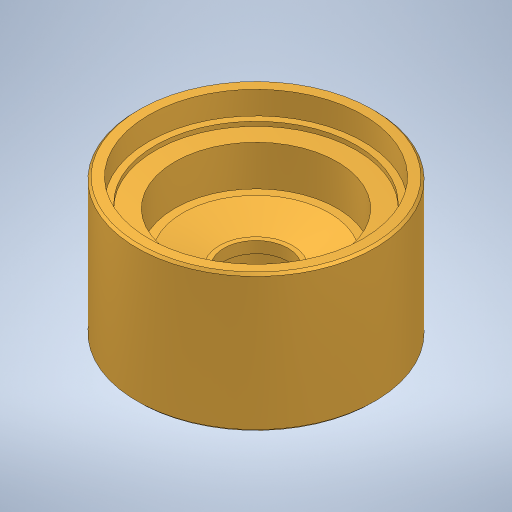
# Autodesk Inventor part: Flywheel
Saved by Autodesk Inventor 2023.2 (Build 272271000, 271)
## iProperties
Created: 2024-02-03
Part Number: Flywheel
Material: Brass, Soft Yellow
Document SubType Name: Modeling
Designer: Nathan Cai
Mass: 186.843 g
Surface Area: 85.7696 cm^2
Volume: 22.0594 cm^3
Density: 8.47 g/cm^3
Appearance: Brass - Satin
Author: Nathan Cai
Autodesk Inventor part; units mm, degrees
ref_plane "YZ Plane" through (0, 0, 0) normal (1, 0, 0) x (0, 1, 0)
ref_plane "XZ Plane" through (0, 0, 0) normal (0, 1, 0) x (-1, 0, 0)
ref_plane "XY Plane" through (0, 0, 0) normal (0, 0, 1) x (1, 0, 0)
sketch "Sketch2" plane through (0, 0, 0) normal (1, 0, 0) x (0, 1, 0)
  line L0 (0, 0) -> (19.05, 0)
  line L1 (19.05, 0) -> (19.05, -6.35)
  line L2 (19.05, -6.35) -> (0, -6.35)
  line L3 (0, -6.35) -> (0, 0)
  line L4 (0, 0) -> (19.05, 0)
  line L5 (19.05, 0) -> (19.05, -20.6375)
  line L6 (19.05, -20.6375) -> (0, -20.6375)
  line L7 (0, -20.6375) -> (0, 0)
  line L8 (0, -16.7624) -> (10.3188, -16.7624) construction
  line L9 (10.3188, -16.7624) -> (10.3188, -6.35)
  line L10 (10.3188, -6.35) -> (0, -6.35)
  line L11 (0, -6.35) -> (0, -16.7624)
  line L12 (10.3188, -16.7624) -> (0, -19.05)
  line L13 (6.35, -20.6375) -> (19.05, -17.4625)
  line L14 (19.05, 0) -> (12.05, 0)
  line L15 (12.05, 0) -> (12.05, -13.975)
  line L16 (12.05, -13.975) -> (19.05, -13.975)
  line L17 (19.05, -13.975) -> (19.05, 0)
  line L18 (10.3188, -15.0812) -> (4.7625, -15.0812)
  line L19 (4.7625, -15.0812) -> (4.7625, -6.35)
  line L20 (4.7625, -6.35) -> (10.3188, -6.35)
  line L21 (10.3188, -6.35) -> (10.3188, -15.0812)
  line L22 (4.7625, -9.525) -> (10.3188, -15.0812)
  line L23 (19.05, 0) -> (23.8125, 0)
  line L24 (23.8125, 0) -> (23.8125, -20.6375)
  line L25 (23.8125, -20.6375) -> (19.05, -20.6375)
  line L26 (19.05, -20.6375) -> (19.05, 0)
  line L27 (23.8125, 0) -> (19.8125, 0)
  line L28 (19.8125, 0) -> (19.8125, -18.5)
  line L29 (19.8125, -18.5) -> (23.8125, -18.5)
  line L30 (23.8125, -18.5) -> (23.8125, 0)
  line L31 (19.8125, -17.4625) -> (19.05, -17.4625)
  line L32 (12.05, -12.7) -> (10.3188, -6.35)
  line L33 (10.3188, -6.35) -> (8.3344, -6.35)
  line L34 (8.3344, -6.35) -> (8.3344, -5.5562)
  line L35 (8.3344, -5.5562) -> (10.3188, -5.5562)
  line L36 (10.3188, -5.5562) -> (10.3188, -6.35)
  point P0 (19.05, -13.975)
  point P1 (12.05, -6.35)
  point P2 (4.7625, -6.35)
  point P3 (12.05, 0)
  point P4 (23.8125, -18.5)
  point P5 (10.3188, -6.35)
  point P6 (10.3188, -6.35)
  dimension "d4" = 19.05
  dimension "d5" = 6.35
  dimension "d6" = 20.6375
  dimension "d7" = 12.5
  dimension "d9" = 10.3187
  dimension "d11" = 19.05
  dimension "d35" = 6.35
  dimension "d36" = 7
  dimension "d37" = 13.975
  dimension "d38" = 17.4625
  dimension "d41" = 4.7625
  dimension "d42" = 5.5563
  dimension "d43" = 3.175
  dimension "d54" = 4.7625
  dimension "d55" = 4
  dimension "d56" = 18.5
  dimension "d57" = 12.7
  dimension "d58" = 1.9844
  dimension "d59" = 0.7937
  constraints: 74 end point, 16 parallel, 14 point on line, 9 perpendicular, 8 horizontal
  measures "d4" distance of L1.end L2.end
  measures "d5" distance of L0.end L1.end
  measures "d6" distance of L4.end L5.end
  measures "d7" angle of L8 L12
  measures "d9" distance between parallel lines of L7 L9
  measures "d11" distance from line of L0 L12.end
  measures "d35" distance from line of L7 L13.start
  measures "d36" distance of L16.end L15.end
  measures "d37" distance of L15.end L14.end
  measures "d38" distance from line of L0 L13.end
  measures "d41" distance between parallel lines of L7 L19
  measures "d42" distance between parallel lines of L6 L18
  measures "d43" distance from line of L10 L22.start
  measures "d54" distance between parallel lines of L26 L24
  measures "d55" distance of L29.end L28.end
  measures "d56" distance between parallel lines of L23 L29
  measures "d57" distance from line of L14 L32.start
  measures "d58" distance of L34.end L35.end
  measures "d59" distance of L33.end L34.end
revolve "Revolution1" add sketch "Sketch2" angle 360 about axis through (0, 0, 0) along (0, 1, 0) contours L2 L9 L22 L19 | L32 L15 L16 L5 L13 L6 L7 L12 L9 | L2 L34 L35 L36 | L28 L29 L24 L25 L5 L31 | L5 L6 L13
chamfer "Chamfer1" distance 0.3969 angle 45 3 edges at (0, 0, 20.6375) (0, 4.7625, 9.525) (0, 23.8125, 20.6375)
thicken "Thicken1" operation cut thickness 0.1 both sides no extend neighbours no toward (0.1604113, 0, -0.9870503) faces at (2.9676, 22.4792, -18.2604)
thicken "Thicken2" operation cut thickness 0.1 both sides no extend neighbours no toward (0.0804666, 0, -0.9967573) faces at (1.1245, 16.7167, -13.9297)
thicken "Thicken3" [suppressed]
thicken "Thicken4" operation add thickness 0.1 both sides no extend neighbours yes toward (0.0804666, 0, -0.9967573) faces at (0.511, 5.9531, -6.3294)
body "Solid2"
